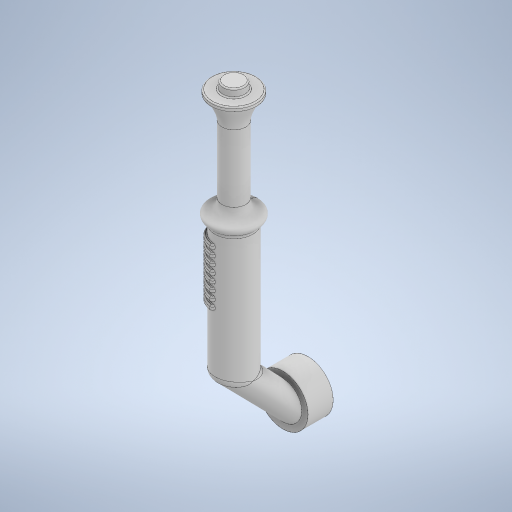
# Autodesk Inventor part: 塔3
Saved by Autodesk Inventor 2024 (Build 280153000, 153)
## iProperties
Created: 2024-05-25
Part Number: 塔3
Material: 一般
Document SubType Name: Modeling
Designer: User
Density: 1 g/cm^3
Appearance: 預設
Author: User
Autodesk Inventor part; units mm, degrees
ref_plane "YZ Plane" through (0, 0, 0) normal (1, 0, 0) x (0, 1, 0)
ref_plane "XY Plane" through (0, 0, 0) normal (0, 0, 1) x (1, 0, 0)
sketch "草圖1" plane through (0, 0, 0) normal (0, 0, 1) x (1, 0, 0)
  circle A0 centre (0, 0) radius 10
  dimension "d0" = 20
  constraints: 1 centre point, 1 coincident
  measures "d0" diameter of A0
extrude "擠出1" add sketch "草圖1" along normal blind 5
sketch "草圖2" plane through (0, 0, 5) normal (0, 0, 1) x (1, 0, 0)
  circle A0 centre (0, 0) radius 7.5
  dimension "d3" = 15
  constraints: 1 centre point, 1 coincident
  measures "d3" diameter of A0
ref_plane "工作平面1" through (0, 20, 0) normal (0, 1, 0) x (-1, 0, 0)
sketch "草圖3" plane through (0, 20, 0) normal (0, 1, 0) x (-1, 0, 0)
  circle A0 centre (0, 24.5124) radius 7.5
  point P0 (0, 0)
  dimension "d5" = 15
  constraints: 1 centre point
  measures "d5" diameter of A0
loft "斷面混成1" add profiles "草圖2", "草圖3"
sketch "草圖4" plane through (0, 20, 24.5124) normal (0, 1, 0) x (1, 0, 0)
  circle A0 centre (0, 0) radius 7.5
  point P0 (0, 24.5124)
  constraints: 1 centre point
extrude "擠出2" add sketch "草圖4" along normal blind 52
fillet "圓角1" radius 3.8 2 edges at (0, 20, 17.0124) (0, 20, 32.0124)
sketch "草圖5" plane through (0, 0, 0) normal (1, 0, 0) x (0, 1, 0)
  line L0 (72, 17.0124) -> (72, 32.0124) projected
  line L1 (72, 24.5124) -> (115, 24.5124)
  line L2 (115, 24.5124) -> (115, 17.0124)
  line L3 (106.2239, 19.7624) -> (79.5239, 19.7624)
  spline S0 degree 3 poles (115, 17.0124) (113.5761, 16.8144) (109.8519, 19.7624) (106.2239, 19.7624) knots 0 0 0 0 1 1 1 1
  spline S1 degree 4 poles (79.5239, 19.7624) (77.9985, 19.7624) (74.3799, 18.9169) (76.5896, 12.6213) (72, 15.5945) (72, 17.0124) knots 0 0 0 0 0 0.511135 1 1 1 1 1
  point P0 (0, 0)
  point P1 (112.376, 17.8784)
  point P2 (75.9658, 17.8033)
  point P3 (74.3849, 14.9973)
  dimension "d13" = 43
  dimension "d14" = 26.7
  dimension "d15" = 4.75
  constraints: 6 end point, 4 horizontal, 1 midpoint, 1 perpendicular, 1 vertical, 7 other
  measures "d13" distance of L1.start L1.end
  measures "d14" distance of L3.start L3.end
  measures "d15" distance between parallel lines of L3 L1
revolve "迴轉1" add sketch "草圖5" angle 360 about axis through (0, 72, 24.5124) along (0, 1, 0)
fillet "圓角2" radius 2 2 edges at (-5.3033, 72, 29.8157) (5.3033, 72, 19.2091)
sketch "草圖6" plane through (0, 115, 24.5124) normal (0, 1, 0) x (1, 0, 0)
  circle A0 centre (0, 0) radius 7.5 projected
  circle A1 centre (0, 0) radius 9
  point P0 (0, 24.5124)
  point P1 (0, 7.5)
  dimension "d18" = 18
  constraints: 1 centre point, 1 coincident, 1 vertical alignment
  measures "d18" diameter of A1
extrude "擠出3" add sketch "草圖6" along normal blind 2 contours A0 | A1
sketch "草圖7" plane through (0, 117, 24.5124) normal (0, 1, 0) x (1, 0, 0)
  circle A0 centre (0, 0) radius 9 projected
  circle A1 centre (0, 0) radius 4.5
  point P0 (0, 24.5124)
  dimension "d21" = 9
  constraints: 1 centre point, 1 coincident
  measures "d21" diameter of A1
extrude "擠出4" add sketch "草圖7" along normal blind 3 draft -5 contours A1
fillet "圓角3" radius 0.5 5 edges at (-4.2375, 120, 24.5124) (-4.5, 117, 24.5124) (-9, 117, 24.5124) (-9, 115, 24.5124) (0, 115, 32.0124)
sketch "草圖8" plane through (0, 0, 0) normal (0, 0, -1) x (-1, 0, 0)
  circle A0 centre (0, 0) radius 10
  constraints: 1 centre point, 1 coincident
extrude "擠出5" add sketch "草圖8" along normal blind 5
sketch "草圖9" plane through (0, 0, 0) normal (1, 0, 0) x (0, 1, 0)
  line L0 (0, 5) -> (20, 24.5124) projected
  line L1 (20, 24.5124) -> (70.6279, 24.5124)
  line L2 (21.5541, 32.0124) -> (70.6279, 32.0124) projected
  line L3 (65.1714, 16.0124) -> (67.1714, 16.0124)
  line L4 (67.1714, 16.0124) -> (67.1714, 33.0124)
  line L5 (67.1714, 33.0124) -> (65.1714, 33.0124)
  line L6 (65.1714, 33.0124) -> (65.1714, 16.0124)
  line L7 (65.1714, 16.0124) -> (67.1714, 33.0124) construction
  line L8 (67.1714, 16.0124) -> (65.1714, 33.0124) construction
  line L9 (64.1714, 16.0124) -> (64.1714, 33.0124)
  line L10 (62.1714, 16.0124) -> (64.1714, 16.0124)
  line L11 (62.1714, 33.0124) -> (62.1714, 16.0124)
  line L12 (64.1714, 33.0124) -> (62.1714, 33.0124)
  line L13 (61.1714, 16.0124) -> (61.1714, 33.0124)
  line L14 (59.1714, 16.0124) -> (61.1714, 16.0124)
  line L15 (59.1714, 33.0124) -> (59.1714, 16.0124)
  line L16 (61.1714, 33.0124) -> (59.1714, 33.0124)
  line L17 (58.1714, 16.0124) -> (58.1714, 33.0124)
  line L18 (56.1714, 16.0124) -> (58.1714, 16.0124)
  line L19 (56.1714, 33.0124) -> (56.1714, 16.0124)
  line L20 (58.1714, 33.0124) -> (56.1714, 33.0124)
  line L21 (55.1714, 16.0124) -> (55.1714, 33.0124)
  line L22 (53.1714, 16.0124) -> (55.1714, 16.0124)
  line L23 (53.1714, 33.0124) -> (53.1714, 16.0124)
  line L24 (55.1714, 33.0124) -> (53.1714, 33.0124)
  line L25 (52.1714, 16.0124) -> (52.1714, 33.0124)
  line L26 (50.1714, 16.0124) -> (52.1714, 16.0124)
  line L27 (50.1714, 33.0124) -> (50.1714, 16.0124)
  line L28 (52.1714, 33.0124) -> (50.1714, 33.0124)
  line L29 (49.1714, 16.0124) -> (49.1714, 33.0124)
  line L30 (47.1714, 16.0124) -> (49.1714, 16.0124)
  line L31 (47.1714, 33.0124) -> (47.1714, 16.0124)
  line L32 (49.1714, 33.0124) -> (47.1714, 33.0124)
  line L33 (46.1714, 16.0124) -> (46.1714, 33.0124)
  line L34 (44.1714, 16.0124) -> (46.1714, 16.0124)
  line L35 (44.1714, 33.0124) -> (44.1714, 16.0124)
  line L36 (46.1714, 33.0124) -> (44.1714, 33.0124)
  point P0 (0, 0)
  point P1 (66.1714, 24.5124)
  point P2 (50.1714, 32.0124)
  point P3 (52.1714, 32.0124)
  point P4 (65.1714, 32.0124)
  point P5 (67.1714, 32.0124)
  point P6 (62.1714, 32.0124)
  point P7 (64.1714, 32.0124)
  point P8 (44.1714, 32.0124)
  point P9 (46.1714, 32.0124)
  point P10 (47.1714, 32.0124)
  point P11 (49.1714, 32.0124)
  point P12 (53.1714, 32.0124)
  point P13 (55.1714, 32.0124)
  point P14 (56.1714, 32.0124)
  point P15 (58.1714, 32.0124)
  point P16 (59.1714, 32.0124)
  point P17 (61.1714, 32.0124)
  dimension "d27" = 2
  dimension "d28" = 17
  dimension "d31" = 3
  constraints: 70 end point, 3 parallel, 2 horizontal, 2 midpoint, 1 perpendicular, 1 point on line, 56 other
  measures "d27" distance of L5.end L4.end
  measures "d28" distance of L4.end L3.end
  measures "d31" distance of L3.end L9.start
revolve "迴轉2" add sketch "草圖9" angle 180 about axis through (0, 20, 24.5124) along (0, -1, 0) contours L35 L36 L33 L2 | L31 L32 L29 L2 | L27 L28 L25 L2 | L23 L24 L21 L2 | L19 L20 L17 L2 | L15 L16 L13 L2 | L11 L12 L9 L2 | L6 L5 L4 L2
fillet "圓角4" radius 1 16 edges at (0, 66.1714, 33.0124) (0, 63.1714, 33.0124) (0, 60.1714, 33.0124) (0, 57.1714, 33.0124) (0, 54.1714, 33.0124) (0, 51.1714, 33.0124) (0, 48.1714, 33.0124) (0, 45.1714, 33.0124) (0, 66.1714, 16.0124) (0, 63.1714, 16.0124) (0, 60.1714, 16.0124) (0, 57.1714, 16.0124) (0, 54.1714, 16.0124) (0, 51.1714, 16.0124) (0, 48.1714, 16.0124) (0, 45.1714, 16.0124)
fillet "圓角5" radius 0.5 48 edges at (-0.3673, 44.1714, 32.7199) (-0.3673, 44.1714, 16.305) (-8.5, 44.1714, 24.5124) (-0.3673, 46.1714, 32.7199) (-0.3673, 46.1714, 16.305) (-8.5, 46.1714, 24.5124) (-0.3673, 47.1714, 32.7199) (-0.3673, 47.1714, 16.305) (-8.5, 47.1714, 24.5124) (-0.3673, 49.1714, 32.7199) (-0.3673, 49.1714, 16.305) (-8.5, 49.1714, 24.5124) (-0.3673, 50.1714, 32.7199) (-0.3673, 50.1714, 16.305) (-8.5, 50.1714, 24.5124) (-0.3673, 52.1714, 32.7199) (-0.3673, 52.1714, 16.305) (-8.5, 52.1714, 24.5124) (-0.3673, 53.1714, 32.7199) (-0.3673, 53.1714, 16.305) (-8.5, 53.1714, 24.5124) (-0.3673, 55.1714, 32.7199) (-0.3673, 55.1714, 16.305) (-8.5, 55.1714, 24.5124) (-0.3673, 56.1714, 32.7199) (-0.3673, 56.1714, 16.305) (-8.5, 56.1714, 24.5124) (-0.3673, 58.1714, 32.7199) (-0.3673, 58.1714, 16.305) (-8.5, 58.1714, 24.5124) (-0.3673, 59.1714, 32.7199) (-0.3673, 59.1714, 16.305) (-8.5, 59.1714, 24.5124) (-0.3673, 61.1714, 32.7199) (-0.3673, 61.1714, 16.305) (-8.5, 61.1714, 24.5124) (-0.3673, 62.1714, 32.7199) (-0.3673, 62.1714, 16.305) (-8.5, 62.1714, 24.5124) (-0.3673, 64.1714, 32.7199) (-0.3673, 64.1714, 16.305) (-8.5, 64.1714, 24.5124) (-0.3673, 65.1714, 16.305) (-0.3673, 65.1714, 32.7199) (-8.5, 65.1714, 24.5124) (-0.3673, 67.1714, 32.7199) (-0.3673, 67.1714, 16.305) (-8.5, 67.1714, 24.5124)
